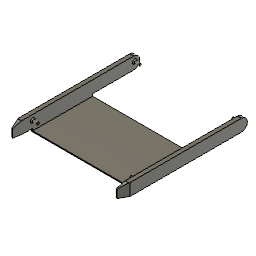
z640-rear-facing (Autodesk Fusion 360 design; units mm, degrees)
Autodesk Fusion 360 part; units mm, degrees
note: some values were not read from the file. Set by a fixed rule: which sketch regions a step uses.
sketch "Sketch1" plane through (0, 0, 0) normal (0, 1, 0) x (1, 0, 0)
  line L0 (0, 0) -> (0, -127)
  line L1 (0, -127) -> (0.8377, -127)
  line L2 (0.8377, -127) -> (4, -117.25)
  line L3 (4, -117.25) -> (4, 0)
  line L4 (4, 0) -> (0, 0)
  dimension "d1" = 127
  dimension "d3" = 117.25
  dimension "d160" = 10.25
  dimension "d182" = 4
  constraint coincident L0.start L4.end
  constraint vertical L0
  constraint perpendicular L0 L1
  constraint perpendicular L1 L3
  constraint perpendicular L0 L4
  measures "d1" distance of L0.start L0.end
  measures "d3" distance of L2.end L3.end
  measures "d160" distance of L1.end L2.end
  measures "d182" distance of L0 L3
extrude "Extrude1" add sketch "Sketch1" along normal blind 12.15
sketch "Sketch3" plane through (0, 0, 0) normal (-1, 0, 0) x (0, 0, 1)
  line L0 (0, 0) -> (127, 0)
  line L1 (127, 0) -> (127, 12.15)
  line L2 (127, 12.15) -> (0, 12.15)
  line L3 (0, 12.15) -> (0, 0)
  line L4 (127, 9.92) -> (118.1878, 12.15)
  line L5 (127, 1.5) -> (116.4057, 0)
  dimension "d11" = 9.09
  dimension "d12" = 2.23
  dimension "d13" = 10.7
  dimension "d14" = 1.5
  constraint coincident L1 L4.start
  constraint coincident L2 L4.end
  constraint coincident L1 L5.start
  constraint coincident L0 L5.end
  measures "d11" distance of L4.start L4.end
  measures "d12" distance of L1.end L4.start
  measures "d13" distance of L5.start L5.end
  measures "d14" distance of L0.end L5.start
extrude "Extrude3" cut sketch "Sketch3" along normal up to surface contours L0 L1 L5 | L1 L2 L4 end surface through (0.8377, 0, 127) normal (-0.95122, 0, -0.308515) offset 0
sketch "Sketch4" plane through (0, 0, 0) normal (-1, 0, 0) x (0, 0, 1)
  line L0 (127, 9.92) -> (118.1878, 12.15)
  line L1 (118.1878, 12.15) -> (0, 12.15)
  line L2 (0, 12.15) -> (0, 0)
  line L3 (0, 0) -> (116.4057, 0)
  line L4 (116.4057, 0) -> (127, 1.5)
  line L5 (127, 1.5) -> (127, 9.92)
  line L6 (0, 6.075) -> (6.075, 6.075)
  circle A0 centre (6.075, 6.075) radius 6.075
  dimension "d17" = 6.075
  constraint midpoint L2 L6.start
  constraint perpendicular L2 L6
  constraint coincident L6.end A0.centre
  constraint coincident L6.start A0
  measures "d17" distance of L6.start L6.end
extrude "Extrude4" cut sketch "Sketch4" against normal up to surface (4 mm away) contours L1 L2 A0 | L2 L3 A0
sketch "Sketch6" plane through (0, 0, 0) normal (0, -1, 0) x (1, 0, 0)
  line L0 (0, 6.075) -> (4, 6.075)
  line L1 (4, 6.075) -> (4, 116.4057)
  line L2 (4, 116.4057) -> (0, 116.4057)
  line L3 (0, 116.4057) -> (0, 6.075)
  line L4 (0, 127) -> (0, 107)
  line L5 (0, 107) -> (0, 47)
  line L6 (0, 47) -> (1, 47)
  line L7 (1, 47) -> (0, 47)
  line L8 (0, 47) -> (0, 107)
  line L9 (0, 107) -> (1, 107)
  line L10 (1, 107) -> (1, 47)
  point P0 (0, 127)
  dimension "d27" = 20
  dimension "d28" = 60
  dimension "d29" = 1
  constraint perpendicular L2 L4
  constraint parallel L3 L5
  constraint perpendicular L5 L6
  constraint horizontal L7
  constraint vertical L8
  constraint horizontal L9
  constraint vertical L10
  constraint coincident P0 L4.start
  measures "d27" distance of P0 L4.end
  measures "d28" distance of L4.end L5.end
  measures "d29" distance of L5.end L6.end
extrude "Extrude6" add sketch "Sketch6" along normal blind 3 contours L3 L5 L6 L7 L8 L9 L10
sketch "Sketch7" plane through (0, 0, 0) normal (-1, 0, 0) x (0, 0, 1)
  arc A0 (6.075, 12.15) -> (6.075, 0) centre (6.075, 6.075) ccw
  line L0 (6.075, 0) -> (47, 0)
  line L1 (47, 0) -> (47, -3)
  line L2 (47, -3) -> (107, -3)
  line L3 (107, -3) -> (107, 0)
  line L4 (107, 0) -> (116.4057, 0)
  line L5 (116.4057, 0) -> (127, 1.5)
  line L6 (127, 1.5) -> (127, 9.92)
  line L7 (127, 9.92) -> (118.1878, 12.15)
  line L8 (118.1878, 12.15) -> (6.075, 12.15)
  line L9 (22, -5.25) -> (43, -5.25)
  line L10 (43, -5.25) -> (43, -1.5)
  line L11 (43, -1.5) -> (22, -1.5)
  line L12 (22, -1.5) -> (22, -5.25)
  line L13 (47, -3) -> (107, -3)
  line L14 (107, -3) -> (107, -2)
  line L15 (107, -2) -> (47, -2)
  line L16 (47, -2) -> (47, -3)
  dimension "d35" = 3.75
  dimension "d36" = 1
  constraint horizontal L9
  constraint vertical L10
  constraint horizontal L11
  constraint vertical L12
  constraint horizontal L13
  constraint vertical L14
  constraint horizontal L15
  constraint vertical L16
  constraint coincident L3 L14.end
  constraint coincident L1.end L2.start
  measures "d35" distance of L9.start L11.end
  measures "d36" distance of L1.end L15.end
extrude "Extrude7" add sketch "Sketch7" along normal blind 51.75 contours L1 L2 L3 L13 L14 L15 L16
sketch "Sketch28" plane through (0, 0, 0) normal (-1, 0, 0) x (0, 0, 1)
  line L0 (116.4057, 0) -> (127, 1.5)
  line L1 (127, 1.5) -> (127, 9.92)
  line L2 (127, 9.92) -> (118.1878, 12.15)
  line L3 (118.1878, 12.15) -> (6.075, 12.15)
  arc A0 (6.075, 12.15) -> (6.075, 0) centre (6.075, 6.075) ccw
  line L4 (116.4057, 0) -> (127, 1.5)
  line L5 (59, -1.5) -> (79, -1.5)
  line L6 (79, 0) -> (116.4057, 0)
  circle A1 centre (106.9086, 6.9514) radius 1.285
  line L7 (127, 7.86) -> (106, 7.86)
  circle A2 centre (5.0436, 6.9514) radius 1.28
  arc A3 (0.45, 3.7804) -> (6.075, 0) centre (6.075, 6.075) ccw
  line L8 (59, 0) -> (59, -1.5)
  line L9 (43, 0) -> (59, 0)
  line L10 (106, 7.86) -> (106, 0)
  line L11 (118.1878, 12.15) -> (6.1, 12.15)
  line L12 (106, 7.86) -> (106.9086, 6.9514)
  line L13 (6.3236, 6.9514) -> (5.0436, 6.9514)
  line L14 (105.6236, 6.9514) -> (106.9086, 6.9514)
  line L15 (127, 1.5) -> (127, 9.92)
  line L16 (127, 9.92) -> (118.1878, 12.15)
  arc A4 (1, 9.4142) -> (0.45, 8.3696) centre (6.075, 6.075) ccw
  line L17 (105.6236, 6.9514) -> (6.3236, 6.9514)
  line L18 (79, -1.5) -> (79, 0)
  line L19 (106, 7.86) -> (107.285, 7.86) construction
  line L20 (43, -1.5) -> (43, 0)
  line L21 (22, -1.5) -> (43, -1.5)
  line L22 (22, 0) -> (22, -1.5)
  line L23 (6.075, 0) -> (22, 0)
  line L24 (47, -2) -> (107, -2)
  line L25 (107, 0) -> (116.4057, 0)
  line L26 (6.075, 0) -> (47, 0)
  line L27 (107, -2) -> (107, 0)
  line L28 (47, 0) -> (47, -2)
  dimension "d168" = 21
  dimension "d169" = 7.86
  dimension "d170" = 1.285
  dimension "d171" = 45
  dimension "d172" = 99.3
  dimension "d173" = 1.28
  constraint perpendicular L7 L15
  constraint coincident L10.end L6
  constraint perpendicular L6 L10
  constraint horizontal L19
  constraint coincident A1.centre L12.end
  constraint coincident L7.end A1
  constraint horizontal L17
  constraint coincident L14.start A1
  constraint coincident L7.start L15
  constraint coincident A2.centre L13.end
  constraint coincident L13.start A2
  constraint parallel L14 L17
  measures "d168" distance of L7.start L7.end
  measures "d169" distance of L7.end L10.end
  measures "d170" distance of L7.end A1.centre
  measures "d171" angle of L12 L19
  measures "d172" distance of L13.start L14.start
  measures "d173" distance of A2.centre L13.start
extrude "Extrude32" add sketch "Sketch28" along normal blind 5.6 contours A1 L7 | A1 L7 L10 L12 L14 | A1 L10 L14 | A1 L10 L14 | L10 L12 L14 | A2
fillet "Fillet15" radius 0.25 2 edges at (-5.6, 6.4867, 105.7106) (-5.6, 6.4885, 3.8503)
mirror "Mirror2" about plane through (-51.75, 0, 0) normal (-1, 0, 0) of bodies 1 merged
fillet "Fillet16" radius 1 4 edges at (0, 7.4142, 3.8503) (0, 7.416, 105.7106) (-103.5, 7.416, 105.7106) (-103.5, 7.4142, 3.8503)
equation "d17 = ( 12.15 / 2 ) * 1 mm"
equation "d37 = ( 103.5 / 2 ) * 1 mm"
equation "d42 = 37.25 mm - 5.5 mm - 2 mm"
equation "d44 = 5.45 mm + 2 mm"
equation "d54 = 35 mm - 3.75 mm"
equation "d141 = 1 mm + 2.25 mm"
equation "d155 = ( 2.57 / 2 ) * 1 mm"
equation "d161 = ( 2.56 / 2 ) * 1 mm"
